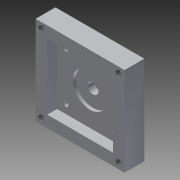
# Autodesk Inventor part: NEMA_17-front
Saved by Autodesk Inventor 2013 (Build 170138000, 138)
## iProperties
Created: 2013-09-16
Part Number: NEMA_17-front
Material: Aluminum 6061
Document SubType Name: Modeling
Designer: Ian
Density: 1 g/cm^3
Author: Ian
Autodesk Inventor part; units mm, degrees
ref_plane "YZ Plane" through (0, 0, 0) normal (1, 0, 0) x (0, 1, 0)
ref_plane "XZ Plane" through (0, 0, 0) normal (0, 1, 0) x (-1, 0, 0)
ref_plane "XY Plane" through (0, 0, 0) normal (0, 0, 1) x (1, 0, 0)
sketch "Sketch1" plane through (0, 0, 0) normal (0, 0, 1) x (1, 0, 0)
  line L0 (-28.575, -28.575) -> (28.575, -28.575)
  line L1 (28.575, -28.575) -> (28.575, 28.575)
  line L2 (28.575, 28.575) -> (-28.575, 28.575)
  line L3 (-28.575, 28.575) -> (-28.575, -28.575)
  line L4 (-28.575, -28.575) -> (28.575, 28.575) construction
  line L5 (28.575, -28.575) -> (-28.575, 28.575) construction
  point P0 (0, 0)
  dimension "d0" = 57.15
  dimension "d1" = 57.15
  constraints: 12 end point, 2 midpoint, 2 parallel, 1 horizontal, 1 perpendicular
  measures "d0" distance of L2.end L1.end
  measures "d1" distance of L1.end L0.end
extrude "Extrusion1" add sketch "Sketch1" along normal blind 12.7
sketch "Sketch2" plane through (0, 0, 12.7) normal (0, 0, 1) x (1, 0, 0)
  line L0 (-21.15, -21.15) -> (21.15, -21.15)
  line L1 (21.15, -21.15) -> (21.15, 21.15)
  line L2 (21.15, 21.15) -> (-21.15, 21.15)
  line L3 (-21.15, 21.15) -> (-21.15, -21.15)
  line L4 (-21.15, -21.15) -> (21.15, 21.15) construction
  line L5 (21.15, -21.15) -> (-21.15, 21.15) construction
  point P0 (0, 0)
  dimension "d4" = 42.3
  dimension "d5" = 42.3
  constraints: 12 end point, 2 midpoint, 2 parallel, 1 horizontal, 1 perpendicular
  measures "d4" distance of L2.end L1.end
  measures "d5" distance of L1.end L0.end
extrude "Extrusion2" cut sketch "Sketch2" against normal blind 6.35
sketch "Sketch3" plane through (0, 0, 0) normal (0, 0, -1) x (-1, 0, 0)
  line L0 (-15.5, -15.5) -> (15.5, -15.5) construction
  line L1 (15.5, -15.5) -> (15.5, 15.5) construction
  line L2 (15.5, 15.5) -> (-15.5, 15.5) construction
  line L3 (-15.5, 15.5) -> (-15.5, -15.5) construction
  line L4 (-15.5, -15.5) -> (15.5, 15.5) construction
  line L5 (15.5, -15.5) -> (-15.5, 15.5) construction
  point P0 (0, 0)
  dimension "d8" = 31
  dimension "d9" = 31
  constraints: 12 end point, 4 coincident, 2 midpoint, 2 parallel, 1 horizontal, 1 perpendicular
  measures "d8" distance of L2.end L1.end
  measures "d9" distance of L1.end L0.end
hole "Hole1" at (15.5, 15.5, 0) at (-15.5, 15.5, 0) at (-15.5, -15.5, 0) at (15.5, -15.5, 0) direction (0, 0, 1) diameter 3.2004 end through all clearance for "Flat Head Machine Screw" size "M3" standard "Ansi Metric M Profile"
sketch "Sketch4" plane through (0, 0, 0) normal (0, 0, -1) x (-1, 0, 0)
  point P0 (0, 0)
  point P1 (0, 0)
  constraints: 1 coincident
sketch "Sketch5" plane through (0, 0, 6.35) normal (0, 0, 1) x (1, 0, 0)
  circle A0 centre (0, 0) radius 11
  dimension "d17" = 22
  constraints: 1 centre point, 1 coincident
  measures "d17" diameter of A0
extrude "Extrusion3" cut sketch "Sketch5" against normal blind 2
hole "Hole2" at (0, 0, 0) direction (0, 0, 1) diameter 7 end through all
sketch "Sketch6" plane through (-28.575, -28.575, 0) normal (0, -1, 0) x (1, 0, 0)
  line L0 (57.15, 0) -> (57.15, 12.7) projected
  line L1 (0, 12.7) -> (57.15, 12.7) projected
  line L2 (0, 0) -> (0, 12.7) projected
  line L3 (28.575, 12.7) -> (28.575, 0) construction
  line L4 (0, 0) -> (57.15, 0) projected
  line L5 (10.16, 4.7625) -> (46.99, 4.7625) construction
  dimension "d27" = 12.7
  dimension "d28" = 10.16
  dimension "d29" = 10.16
  dimension "d45" = 7.9375
  constraints: 4 end point, 1 midpoint, 1 parallel
  measures "d27" distance of L2.start L1.start
  measures "d28" distance from line of L2 L5.start
  measures "d29" distance from line of L0 L5.end
  measures "d45" distance between parallel lines of L1 L5
hole "Hole3" at (-18.415, -28.575, 4.7625) at (18.415, -28.575, 4.7625) direction (0, 1, 0) diameter 4.3434 depth 6.35 tip angle 118 thread size "12-24 UNC" class "2B" standard "ANSI Unified Screw Threads"
sketch "Sketch7" plane through (0, 0, 12.7) normal (0, 0, 1) x (1, 0, 0)
  line L0 (-21.15, 21.15) -> (21.15, 21.15) projected
  line L1 (-28.575, -28.575) -> (28.575, -28.575) projected
  line L2 (28.575, 28.575) -> (-28.575, 28.575) projected
  line L3 (28.575, -28.575) -> (-28.575, 28.575) construction
  line L4 (28.575, 28.575) -> (-28.575, -28.575) construction
  line L5 (0, 28.575) -> (0, 21.15) construction
  line L6 (0, 24.8625) -> (24.8625, 24.8625) construction
  line L7 (-24.8625, -24.8625) -> (24.8625, -24.8625) construction
  line L8 (24.8625, -24.8625) -> (24.8625, 24.8625) construction
  line L9 (24.8625, 24.8625) -> (-24.8625, 24.8625) construction
  line L10 (-24.8625, 24.8625) -> (-24.8625, -24.8625) construction
  line L11 (-24.8625, -24.8625) -> (24.8625, 24.8625) construction
  line L12 (24.8625, -24.8625) -> (-24.8625, 24.8625) construction
  point P0 (0, 0)
  constraints: 20 end point, 5 midpoint, 4 coincident, 3 perpendicular, 2 parallel, 2 point on line, 1 horizontal
hole "Hole4" at (-24.8625, 24.8625, 12.7) at (24.8625, 24.8625, 12.7) at (24.8625, -24.8625, 12.7) at (-24.8625, -24.8625, 12.7) direction (0, 0, -1) diameter 3.9624 depth 5.588 tip angle 118 thread size "10-32 UNF" class "2B" standard "ANSI Unified Screw Threads"
equation "\"d29\" = d28"
body "Solid1"
